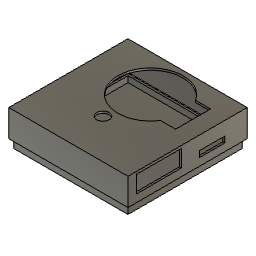
matek_f405_wte_usb_enclosure (Autodesk Fusion 360 design; units mm, degrees)
Autodesk Fusion 360 part; units mm, degrees
note: some values were not read from the file. Set by a fixed rule: which sketch regions a step uses.
sketch "Sketch1" plane through (0, 0, 0) normal (0, 0, 1) x (1, 0, 0)
  line L0 (0, 0) -> (22, 0) construction
  line L1 (22, 0) -> (22, 22) construction
  line L2 (22, 22) -> (0, 22) construction
  line L3 (0, 22) -> (0, 0) construction
  line L4 (22.4, -0.4) -> (22.4, 22.4) construction
  line L5 (22.4, 22.4) -> (-0.4, 22.4) construction
  line L6 (-0.4, 22.4) -> (-0.4, -0.4) construction
  line L7 (-0.4, -0.4) -> (22.4, -0.4) construction
  circle A0 centre (11, 15.5) radius 6.5
  line L8 (16.4772, 19) -> (19.5, 19)
  line L9 (19.5, 19) -> (19.5, 12)
  line L10 (19.5, 12) -> (16.4772, 12)
  line L11 (16.4772, 12) -> (16.4772, 19)
  line L12 (-0.5, 22.5) -> (-0.5, -0.5)
  line L13 (-0.5, -0.5) -> (22.5, -0.5)
  line L14 (22.5, -0.5) -> (22.5, 22.5)
  line L15 (22.5, 22.5) -> (-0.5, 22.5)
  line L16 (-0.9, -0.9) -> (22.9, -0.9)
  line L17 (22.9, -0.9) -> (22.9, 22.9)
  line L18 (22.9, 22.9) -> (-0.9, 22.9)
  line L19 (-0.9, 22.9) -> (-0.9, -0.9)
  dimension "d1" = 22
  dimension "d2" = 22
  dimension "d3" = 0.4
  dimension "d4" = 13
  dimension "d5" = 11
  dimension "d6" = 8.5
  dimension "d7" = 7
  dimension "d37" = 0.5
  dimension "d38" = 0.9
  constraint horizontal L0
  constraint vertical L1
  constraint horizontal L2
  constraint vertical L3
  constraint coincident L0.start L3.end
  constraint tangent L2 A0
  constraint horizontal L8
  constraint vertical L9
  constraint horizontal L10
  constraint vertical L11
  constraint coincident A0 L8.start
  constraint coincident A0 L10.end
  measures "d1" distance of L0.start L2.end
  measures "d2" distance of L0.start L0.end
  measures "d4" diameter of A0
  measures "d5" distance of L3 A0.centre
  measures "d6" distance of A0.centre L9
  measures "d7" distance of L8 L10
extrude "Extrude1" add sketch "Sketch1" along normal blind 0.4 contours L12 L13 L14 L15 | L16 L17 L18 L19 makes body 1
extrude "Extrude2" add sketch "Sketch1" against normal blind 5 contours L16 L17 L18 L19 bodies 1
sketch "Sketch2" plane through (-0.9, 0, 0) normal (-1, 0, 0) x (0, -1, 0)
  line L0 (0.4, -3.5) -> (0.4, 0)
  line L1 (-22.4, 0) -> (-22.4, -3.5)
  line L2 (-22.4, -3.5) -> (0.4, -3.5)
  line L3 (-15.4, -3.5) -> (-6.6, -3.5)
  line L4 (-6.6, -3.5) -> (-6.6, -0.5)
  line L5 (-6.6, -0.5) -> (-15.4, -0.5)
  line L6 (-15.4, -0.5) -> (-15.4, -3.5)
  line L7 (0.4, 0) -> (-22.4, 0)
  line L8 (0.9, -5) -> (0.9, 0.4)
  line L9 (0.9, 0.4) -> (-22.9, 0.4)
  line L10 (-22.9, 0.4) -> (-22.9, -5)
  line L11 (-22.9, -5) -> (0.9, -5)
  dimension "d12" = 7
  dimension "d13" = 7
  dimension "d14" = 3
  constraint horizontal L3
  constraint vertical L4
  constraint horizontal L5
  constraint vertical L6
  constraint coincident L2 L3.start
  measures "d12" distance of L1 L6
  measures "d13" distance of L0 L4
  measures "d14" distance of L3 L5
extrude "Extrude3" cut sketch "Sketch2" against normal blind 0.4 contours L2 L3 L4 L5 L6 bodies 1
sketch "Sketch3" plane through (22.9, 0, 0) normal (1, 0, 0) x (0, 1, 0)
  line L0 (22.4, -3.5) -> (22.4, 0)
  line L1 (-0.4, 0) -> (-0.4, -3.5)
  line L2 (-0.4, -3.5) -> (22.4, -3.5)
  line L3 (0.8, -3.5) -> (9.8, -3.5)
  line L4 (9.8, -3.5) -> (9.8, -0.1)
  line L5 (9.8, -0.1) -> (0.8, -0.1)
  line L6 (0.8, -0.1) -> (0.8, -3.5)
  line L7 (22.4, 0) -> (-0.4, 0)
  line L8 (22.9, -5) -> (22.9, 0.4)
  line L9 (22.9, 0.4) -> (-0.9, 0.4)
  line L10 (-0.9, 0.4) -> (-0.9, -5)
  line L11 (-0.9, -5) -> (22.9, -5)
  dimension "d17" = 9
  dimension "d18" = 3.4
  dimension "d19" = 1.2
  constraint horizontal L3
  constraint vertical L4
  constraint horizontal L5
  constraint vertical L6
  constraint coincident L2 L3.start
  measures "d17" distance of L4 L6
  measures "d18" distance of L3.end L4.end
  measures "d19" distance of L1 L6
extrude "Extrude4" cut sketch "Sketch3" against normal up to surface (0.4 mm away) contours L2 L3 L4 L5 L6 bodies 1
sketch "Sketch4" plane through (22.9, 0, 0) normal (1, 0, 0) x (0, 1, 0)
  line L0 (9.8, -0.1) -> (9.8, -3.5)
  line L1 (9.8, -3.5) -> (22.4, -3.5)
  line L2 (22.4, -3.5) -> (22.4, 0)
  line L3 (-0.4, 0) -> (-0.4, -3.5)
  line L4 (-0.4, -3.5) -> (0.8, -3.5)
  line L5 (0.8, -3.5) -> (0.8, -0.1)
  line L6 (0.8, -0.1) -> (9.8, -0.1)
  line L7 (18.4, -3.5) -> (13.4, -3.5)
  line L8 (13.4, -3.5) -> (13.4, -2.3)
  line L9 (13.4, -2.3) -> (18.4, -2.3)
  line L10 (18.4, -2.3) -> (18.4, -3.5)
  line L11 (22.4, 0) -> (-0.4, 0)
  line L12 (9.8, -0.1) -> (9.8, -3.5)
  line L13 (-0.9, -5) -> (22.9, -5)
  line L14 (22.9, -5) -> (22.9, 0.4)
  line L15 (22.9, 0.4) -> (-0.9, 0.4)
  line L16 (-0.9, 0.4) -> (-0.9, -5)
  line L17 (0.8, -3.5) -> (0.8, -0.1)
  line L18 (0.8, -0.1) -> (9.8, -0.1)
  line L19 (9.8, -3.5) -> (0.8, -3.5)
  dimension "d22" = 4
  dimension "d23" = 5
  dimension "d24" = 1.2
  constraint horizontal L7
  constraint vertical L8
  constraint horizontal L9
  constraint vertical L10
  constraint coincident L1 L7.start
  measures "d22" distance of L2 L10
  measures "d23" distance of L8.end L9.end
  measures "d24" distance of L7.start L9.end
extrude "Extrude5" cut sketch "Sketch4" against normal up to surface (0.4 mm away) contours L1 L7 L8 L9 L10 bodies 1
ref_plane "WorkPlane1" through (11, 11, -5.1) normal (0, 0, -1) x (-1, 0, 0)
sketch "Sketch5" plane through (11, 11, -5.1) normal (0, 0, -1) x (-1, 0, 0)
  line L0 (-11, -11) -> (-11, 11)
  line L1 (-11, 11) -> (11, 11)
  line L2 (-11.4, 11.4) -> (11.4, 11.4)
  line L3 (-11.4, -11.4) -> (-11.4, 11.4)
  line L4 (11.4, 11.4) -> (11.4, -11.4)
  line L5 (11, 11) -> (11, -11)
  line L6 (11, -11) -> (-11, -11)
  line L7 (11.4, -11.4) -> (-11.4, -11.4)
extrude "Extrude6" add sketch "Sketch5" along normal blind 1.2 separate body makes body 2
sketch "Sketch6" plane through (0, 0, -6.3) normal (0, 0, -1) x (1, 0, 0)
  line L0 (0, -22) -> (0, 0)
  line L1 (0, 0) -> (22, 0)
  line L2 (22, 0) -> (22, -22)
  line L3 (22, -22) -> (0, -22)
  line L4 (-0.4, 0.4) -> (-0.4, -22.4)
  line L5 (-0.4, -22.4) -> (22.4, -22.4)
  line L6 (22.4, -22.4) -> (22.4, 0.4)
  line L7 (22.4, 0.4) -> (-0.4, 0.4)
extrude "Extrude7" add sketch "Sketch6" along normal blind 0.4 contours L0 L1 L2 L3 | L4 L5 L6 L7 bodies 2
sketch "Sketch7" plane through (0, 0, 0.4) normal (0, 0, 1) x (-1, 0, 0)
  arc A0 (-16.4772, -19) -> (-16.4772, -12) centre (-11, -15.5) ccw
  line L0 (-16.4772, -19) -> (-19.5, -19)
  line L1 (-19.5, -19) -> (-19.5, -12)
  line L2 (-19.5, -12) -> (-16.4772, -12)
  circle A1 centre (-10, -7) radius 1.25
  line L3 (0.9, -22.9) -> (0.9, 0.9)
  line L4 (0.9, 0.9) -> (-22.9, 0.9)
  line L5 (-22.9, 0.9) -> (-22.9, -22.9)
  line L6 (-22.9, -22.9) -> (0.9, -22.9)
  dimension "d34" = 2.5
  measures "d34" diameter of A1
extrude "Extrude8" cut sketch "Sketch7" against normal up to surface (0.4 mm away) contours A1 bodies 1
named bodies: "matek_usb_enclosure_bottom", "matek_usb_enclosure_top"
